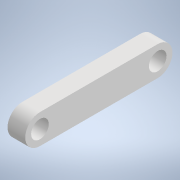
# Autodesk Inventor part: mid joint
Saved by Autodesk Inventor 2020 (Build 240168000, 168)
## iProperties
Created: 2021-11-26
Part Number: mid joint
Material: Generic
Document SubType Name: Modeling
Designer: rwte
Density: 1 g/cm^3
Appearance: Default
Author: rwte
Autodesk Inventor part; units mm, degrees
ref_plane "YZ Plane" through (0, 0, 0) normal (1, 0, 0) x (0, 1, 0)
ref_plane "XZ Plane" through (0, 0, 0) normal (0, 1, 0) x (-1, 0, 0)
ref_plane "XY Plane" through (0, 0, 0) normal (0, 0, 1) x (1, 0, 0)
sketch "Sketch1" plane through (0, 0, 0) normal (1, 0, 0) x (0, 1, 0)
  line L0 (2.5, -10) -> (-2.5, -10) construction
  line L1 (-2.5, -10) -> (-2.5, 10)
  line L2 (-2.5, 10) -> (2.5, 10) construction
  line L3 (2.5, 10) -> (2.5, -10)
  line L4 (2.5, -10) -> (-2.5, 10) construction
  line L5 (-2.5, -10) -> (2.5, 10) construction
  arc A0 (2.5, 10) -> (-2.5, 10) centre (0, 10) ccw
  arc A1 (-2.5, -10) -> (2.5, -10) centre (0, -10) ccw
  circle A2 centre (0, 10) radius 1.5
  circle A3 centre (0, -10) radius 1.5
  point P0 (0, 0)
  dimension "d0" = 5
  dimension "d1" = 20
  dimension "d2" = 3
  dimension "d3" = 3
  constraints: 12 end point, 4 centre point, 4 midpoint, 4 point on circle, 2 coincident, 2 parallel, 1 horizontal, 1 perpendicular
  measures "d0" distance of L1.end L2.end
  measures "d1" distance of L0.end L1.end
  measures "d2" diameter of A2
  measures "d3" diameter of A3
extrude "Extrusion1" add sketch "Sketch1" along normal mid plane 3
body "Solid1"
